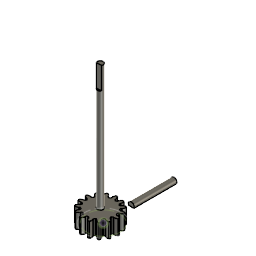
axle (Autodesk Fusion 360 design; units mm, degrees)
part number: 2026-05-16-01-15-47-219
Autodesk Fusion 360 part; units mm, degrees
note: some values were not read from the file. Chosen so that the rebuilt part matches the saved one: which bodies a step acts on; which pieces of a blend or face edit are solid. Set by a fixed rule: which sketch regions a step uses.
(part 1 of 4)
sketch "Sketch1" plane through (0, 0, 0) normal (0, 0, 1) x (1, 0, 0)
  circle A0 centre (0, 0) radius 12.5 construction
  dimension "d1" = 25
  constraint coincident A0.centre origin
  measures "d1" diameter of A0
sketch "Base Circle" plane through (0, 0, 0) normal (0, 0, 1) x (1, 0, 0)
  circle A0 centre (0, 0) radius 9.3279
  circle A1 centre (0, 0) radius 1.15
extrude "Extrude1" add sketch "Base Circle" along normal blind 10 makes body 1
sketch "Gear Tooth" plane through (0, 0, 0) normal (0, 0, 1) x (1, 0, 0)
  spline S0 degree 5 poles (10.2902, -1.2369) (10.2964, -1.2376) (10.3089, -1.2389) (10.3277, -1.2404) (10.3528, -1.2412) (10.3842, -1.2409) (10.4157, -1.2395) (10.4473, -1.2374) (10.4789, -1.2351) (10.5106, -1.2325) (10.5422, -1.2296) (10.5739, -1.2264) (10.6056, -1.2228) (10.6373, -1.2187) (10.6691, -1.2141) (10.7008, -1.209) (10.7326, -1.2035) (10.7644, -1.1976) (10.7962, -1.1915) (10.828, -1.1851) (10.8597, -1.1784) (10.8915, -1.1714) (10.9233, -1.1641) (10.9551, -1.1564) (10.9869, -1.1485) (11.0187, -1.1402) (11.0505, -1.1317) (11.0823, -1.1229) (11.114, -1.1138) (11.1458, -1.1044) (11.1776, -1.0948) (11.2093, -1.085) (11.241, -1.0748) (11.2727, -1.0645) (11.3045, -1.0538) (11.3361, -1.0429) (11.3678, -1.0318) (11.3995, -1.0204) (11.4311, -1.0087) (11.4627, -0.9969) (11.4943, -0.9847) (11.5259, -0.9724) (11.5575, -0.9598) (11.589, -0.947) (11.6206, -0.934) (11.6521, -0.9207) (11.6835, -0.9072) (11.715, -0.8935) (11.7464, -0.8796) (11.7778, -0.8654) (11.8091, -0.8511) (11.8405, -0.8365) (11.8718, -0.8217) (11.9031, -0.8067) (11.9343, -0.7914) (11.9655, -0.776) (11.9967, -0.7603) (12.0279, -0.7445) (12.059, -0.7284) (12.0901, -0.7122) (12.1211, -0.6957) (12.1521, -0.679) (12.1831, -0.6622) (12.214, -0.6451) (12.2449, -0.6278) (12.2758, -0.6103) (12.3066, -0.5927) (12.3374, -0.5748) (12.3682, -0.5567) (12.3988, -0.5385) (12.4295, -0.52) (12.454, -0.5051) (12.4723, -0.4939) (12.4846, -0.4863) (12.4907, -0.4825) knots 0 0 0 0 0 0 0.01428571 0.02857143 0.04285714 0.05714286 0.07142857 0.08571429 0.1 0.11428571 0.12857143 0.14285714 0.15714286 0.17142857 0.18571429 0.2 0.21428571 0.22857143 0.24285714 0.25714286 0.27142857 0.28571429 0.3 0.31428571 0.32857143 0.34285714 0.35714286 0.37142857 0.38571429 0.4 0.41428571 0.42857143 0.44285714 0.45714286 0.47142857 0.48571429 0.5 0.51428571 0.52857143 0.54285714 0.55714286 0.57142857 0.58571429 0.6 0.61428571 0.62857143 0.64285714 0.65714286 0.67142857 0.68571429 0.7 0.71428571 0.72857143 0.74285714 0.75714286 0.77142857 0.78571429 0.8 0.81428571 0.82857143 0.84285714 0.85714286 0.87142857 0.88571429 0.9 0.91428571 0.92857143 0.94285714 0.95714286 0.97142857 0.98571429 1 1 1 1 1 1
  spline S1 degree 5 poles (10.2902, 1.2369) (10.2964, 1.2376) (10.3089, 1.2389) (10.3277, 1.2404) (10.3528, 1.2412) (10.3842, 1.2409) (10.4157, 1.2395) (10.4473, 1.2374) (10.4789, 1.2351) (10.5106, 1.2325) (10.5422, 1.2296) (10.5739, 1.2264) (10.6056, 1.2228) (10.6373, 1.2187) (10.6691, 1.2141) (10.7008, 1.209) (10.7326, 1.2035) (10.7644, 1.1976) (10.7962, 1.1915) (10.828, 1.1851) (10.8597, 1.1784) (10.8915, 1.1714) (10.9233, 1.1641) (10.9551, 1.1564) (10.9869, 1.1485) (11.0187, 1.1402) (11.0505, 1.1317) (11.0823, 1.1229) (11.114, 1.1138) (11.1458, 1.1044) (11.1776, 1.0948) (11.2093, 1.085) (11.241, 1.0748) (11.2727, 1.0645) (11.3045, 1.0538) (11.3361, 1.0429) (11.3678, 1.0318) (11.3995, 1.0204) (11.4311, 1.0087) (11.4627, 0.9969) (11.4943, 0.9847) (11.5259, 0.9724) (11.5575, 0.9598) (11.589, 0.947) (11.6206, 0.934) (11.6521, 0.9207) (11.6835, 0.9072) (11.715, 0.8935) (11.7464, 0.8796) (11.7778, 0.8654) (11.8091, 0.8511) (11.8405, 0.8365) (11.8718, 0.8217) (11.9031, 0.8067) (11.9343, 0.7914) (11.9655, 0.776) (11.9967, 0.7603) (12.0279, 0.7445) (12.059, 0.7284) (12.0901, 0.7122) (12.1211, 0.6957) (12.1521, 0.679) (12.1831, 0.6622) (12.214, 0.6451) (12.2449, 0.6278) (12.2758, 0.6103) (12.3066, 0.5927) (12.3374, 0.5748) (12.3682, 0.5567) (12.3988, 0.5385) (12.4295, 0.52) (12.454, 0.5051) (12.4723, 0.4939) (12.4846, 0.4863) (12.4907, 0.4825) knots 0 0 0 0 0 0 0.01428571 0.02857143 0.04285714 0.05714286 0.07142857 0.08571429 0.1 0.11428571 0.12857143 0.14285714 0.15714286 0.17142857 0.18571429 0.2 0.21428571 0.22857143 0.24285714 0.25714286 0.27142857 0.28571429 0.3 0.31428571 0.32857143 0.34285714 0.35714286 0.37142857 0.38571429 0.4 0.41428571 0.42857143 0.44285714 0.45714286 0.47142857 0.48571429 0.5 0.51428571 0.52857143 0.54285714 0.55714286 0.57142857 0.58571429 0.6 0.61428571 0.62857143 0.64285714 0.65714286 0.67142857 0.68571429 0.7 0.71428571 0.72857143 0.74285714 0.75714286 0.77142857 0.78571429 0.8 0.81428571 0.82857143 0.84285714 0.85714286 0.87142857 0.88571429 0.9 0.91428571 0.92857143 0.94285714 0.95714286 0.97142857 0.98571429 1 1 1 1 1 1
  arc A0 (12.4907, -0.4825) -> (12.4907, 0.4825) centre (0, 0) ccw
  line L0 (9.2514, -1.112) -> (10.2902, -1.2369)
  line L1 (9.2514, 1.112) -> (10.2902, 1.2369)
  line L2 (9.2514, -1.112) -> (9.2514, 1.112)
  point P0 (10.4437, -1.2376)
  point P1 (10.599, -1.2235)
  point P2 (10.7553, -1.1992)
  point P3 (10.9123, -1.1666)
  point P4 (11.0699, -1.1263)
  point P5 (11.2278, -1.079)
  point P6 (11.3861, -1.0252)
  point P7 (11.5444, -0.965)
  point P8 (11.7028, -0.8988)
  point P9 (11.861, -0.8267)
  point P10 (12.019, -0.749)
  point P11 (12.1767, -0.6656)
  point P12 (12.334, -0.5768)
  point P13 (10.4437, 1.2376)
  point P14 (10.599, 1.2235)
  point P15 (10.7553, 1.1992)
  point P16 (10.9123, 1.1666)
  point P17 (11.0699, 1.1263)
  point P18 (11.2278, 1.079)
  point P19 (11.3861, 1.0252)
  point P20 (11.5444, 0.965)
  point P21 (11.7028, 0.8988)
  point P22 (11.861, 0.8267)
  point P23 (12.019, 0.749)
  point P24 (12.1767, 0.6656)
  point P25 (12.334, 0.5768)
extrude "Extrude2" add sketch "Gear Tooth" along normal blind 10 bodies 1
fillet "Fillet1" radius 0.8 2 edges at (9.2613, -1.1132, 5) (9.2613, 1.1132, 5) on bodies 1
pattern_circular "C-Pattern1" count 15 over 360 about axis through (0, 0, 0) along (0, 0, 1) of "Extrude2", "Fillet1"
sketch "Diametrial Pitch Circle" plane through (0, 0, 0) normal (0, 0, 1) x (1, 0, 0)
  circle A0 centre (0, 0) radius 11.0294 construction
sketch "Sketch5" plane through (0, 0, 0) normal (0, 0, 1) x (1, 0, 0)
  circle A0 centre (0, 0) radius 1.15
  dimension "d10" = 2.3
  constraint coincident A0.centre origin
  measures "d10" diameter of A0
extrude "Extrude3" add sketch "Sketch5" along normal blind 10 bodies 1
sketch "Sketch6" plane through (0, 0, 0) normal (0, 0, 1) x (1, 0, 0)
  circle A0 centre (0, 0) radius 2
  line L0 (1.7319, -1.0003) -> (-1.7676, -0.9358)
  dimension "d13" = 4
  dimension "d14" = 3.5
  constraint coincident A0.centre origin
  constraint coincident A0 L0.start
  constraint coincident A0 L0.end
  measures "d13" diameter of A0
  measures "d14" distance of L0.start L0.end
move_body "Move1" bodies 1 to x (1, 0, 0) y (0, 1, 0) z (0, 0, 1) at (0, 0, 80)
extrude "Extrude4" add sketch "Sketch6" along normal blind 80 bodies 1
extrude "Extrude5" cut sketch "Sketch6" along normal blind 15 contours A0 L0 picked at (-0.551, -1.0376) bodies 1
move_body "Move2" bodies 1 to x (1, 0, 0) y (0, -1, 0) z (0, 0, -1) at (0, 0.0546, 170)
extrude "Extrude6" add sketch "Sketch6" along normal blind 80 bodies 1
extrude "Extrude7" cut sketch "Sketch6" along normal blind 15 contours A0 L0 picked at (-0.551, -1.0376) bodies 1
move_body "Move3" bodies 1 to x (1, 0, 0) y (0, 0, 1) z (0, -1, 0) at (0, 0, 0)
move_body "Move4" bodies 1 to x (1, 0, 0) y (0, 1, 0) z (0, 0, 1) at (0, 85, 0)
move_body "Move5" bodies 1 to x (1, 0, 0) y (0, 1, 0) z (0, 0, 1) at (0, 0, 13)
sketch "Sketch7" plane through (0, 5, 0) normal (0, 1, 0) x (-1, 0, 0)
  circle A0 centre (0, 13) radius 2
  arc A1 (-9.1027, 15.0919) -> (-9.1444, 14.8959) centre (0, 13.0546) ccw
  arc A2 (-10.0241, 14.2595) -> (-9.1444, 14.8959) centre (-9.9287, 15.0538) ccw
  line L0 (-10.0241, 14.2595) -> (-10.2902, 14.2915)
  spline S0 degree 5 poles (-10.2902, 14.2915) (-10.2964, 14.2922) (-10.3089, 14.2935) (-10.3277, 14.295) (-10.3528, 14.2958) (-10.3842, 14.2955) (-10.4157, 14.2941) (-10.4473, 14.2921) (-10.4789, 14.2897) (-10.5106, 14.2871) (-10.5422, 14.2842) (-10.5739, 14.281) (-10.6056, 14.2774) (-10.6373, 14.2733) (-10.6691, 14.2687) (-10.7008, 14.2636) (-10.7326, 14.2581) (-10.7644, 14.2522) (-10.7962, 14.2461) (-10.828, 14.2397) (-10.8597, 14.233) (-10.8915, 14.226) (-10.9233, 14.2187) (-10.9551, 14.211) (-10.9869, 14.2031) (-11.0187, 14.1948) (-11.0505, 14.1863) (-11.0823, 14.1775) (-11.114, 14.1684) (-11.1458, 14.1591) (-11.1776, 14.1494) (-11.2093, 14.1396) (-11.241, 14.1295) (-11.2727, 14.1191) (-11.3045, 14.1084) (-11.3361, 14.0975) (-11.3678, 14.0864) (-11.3995, 14.075) (-11.4311, 14.0633) (-11.4627, 14.0515) (-11.4943, 14.0394) (-11.5259, 14.027) (-11.5575, 14.0144) (-11.589, 14.0016) (-11.6206, 13.9886) (-11.6521, 13.9753) (-11.6835, 13.9618) (-11.715, 13.9481) (-11.7464, 13.9342) (-11.7778, 13.92) (-11.8091, 13.9057) (-11.8405, 13.8911) (-11.8718, 13.8763) (-11.9031, 13.8613) (-11.9343, 13.846) (-11.9655, 13.8306) (-11.9967, 13.815) (-12.0279, 13.7991) (-12.059, 13.783) (-12.0901, 13.7668) (-12.1211, 13.7503) (-12.1521, 13.7336) (-12.1831, 13.7168) (-12.214, 13.6997) (-12.2449, 13.6824) (-12.2758, 13.6649) (-12.3066, 13.6473) (-12.3374, 13.6294) (-12.3682, 13.6113) (-12.3988, 13.5931) (-12.4295, 13.5746) (-12.454, 13.5597) (-12.4723, 13.5485) (-12.4846, 13.5409) (-12.4907, 13.5371) knots 0 0 0 0 0 0 0.01428571 0.02857143 0.04285714 0.05714286 0.07142857 0.08571429 0.1 0.11428571 0.12857143 0.14285714 0.15714286 0.17142857 0.18571429 0.2 0.21428571 0.22857143 0.24285714 0.25714286 0.27142857 0.28571429 0.3 0.31428571 0.32857143 0.34285714 0.35714286 0.37142857 0.38571429 0.4 0.41428571 0.42857143 0.44285714 0.45714286 0.47142857 0.48571429 0.5 0.51428571 0.52857143 0.54285714 0.55714286 0.57142857 0.58571429 0.6 0.61428571 0.62857143 0.64285714 0.65714286 0.67142857 0.68571429 0.7 0.71428571 0.72857143 0.74285714 0.75714286 0.77142857 0.78571429 0.8 0.81428571 0.82857143 0.84285714 0.85714286 0.87142857 0.88571429 0.9 0.91428571 0.92857143 0.94285714 0.95714286 0.97142857 0.98571429 1 1 1 1 1 1
  arc A3 (-12.4907, 13.5371) -> (-12.4907, 12.5721) centre (0, 13.0546) ccw
  spline S1 degree 5 poles (-12.4907, 12.5721) (-12.4846, 12.5683) (-12.4723, 12.5608) (-12.454, 12.5495) (-12.4295, 12.5346) (-12.3988, 12.5161) (-12.3682, 12.4979) (-12.3374, 12.4798) (-12.3066, 12.4619) (-12.2758, 12.4443) (-12.2449, 12.4268) (-12.214, 12.4095) (-12.1831, 12.3925) (-12.1521, 12.3756) (-12.1211, 12.3589) (-12.0901, 12.3424) (-12.059, 12.3262) (-12.0279, 12.3101) (-11.9967, 12.2943) (-11.9655, 12.2786) (-11.9343, 12.2632) (-11.9031, 12.2479) (-11.8718, 12.2329) (-11.8405, 12.2181) (-11.8091, 12.2035) (-11.7778, 12.1892) (-11.7464, 12.175) (-11.715, 12.1611) (-11.6835, 12.1474) (-11.6521, 12.1339) (-11.6206, 12.1206) (-11.589, 12.1076) (-11.5575, 12.0948) (-11.5259, 12.0822) (-11.4943, 12.0699) (-11.4627, 12.0578) (-11.4311, 12.0459) (-11.3995, 12.0342) (-11.3678, 12.0229) (-11.3361, 12.0117) (-11.3045, 12.0008) (-11.2727, 11.9902) (-11.241, 11.9798) (-11.2093, 11.9696) (-11.1776, 11.9598) (-11.1458, 11.9502) (-11.114, 11.9408) (-11.0823, 11.9317) (-11.0505, 11.9229) (-11.0187, 11.9144) (-10.9869, 11.9061) (-10.9551, 11.8982) (-10.9233, 11.8905) (-10.8915, 11.8832) (-10.8597, 11.8762) (-10.828, 11.8696) (-10.7962, 11.8631) (-10.7644, 11.857) (-10.7326, 11.8512) (-10.7008, 11.8457) (-10.6691, 11.8406) (-10.6373, 11.8359) (-10.6056, 11.8318) (-10.5739, 11.8282) (-10.5422, 11.825) (-10.5106, 11.8222) (-10.4789, 11.8195) (-10.4473, 11.8172) (-10.4157, 11.8151) (-10.3842, 11.8138) (-10.3528, 11.8134) (-10.3277, 11.8143) (-10.3089, 11.8157) (-10.2964, 11.817) (-10.2902, 11.8177) knots -1 -1 -1 -1 -1 -1 -0.98571429 -0.97142857 -0.95714286 -0.94285714 -0.92857143 -0.91428571 -0.9 -0.88571429 -0.87142857 -0.85714286 -0.84285714 -0.82857143 -0.81428571 -0.8 -0.78571429 -0.77142857 -0.75714286 -0.74285714 -0.72857143 -0.71428571 -0.7 -0.68571429 -0.67142857 -0.65714286 -0.64285714 -0.62857143 -0.61428571 -0.6 -0.58571429 -0.57142857 -0.55714286 -0.54285714 -0.52857143 -0.51428571 -0.5 -0.48571429 -0.47142857 -0.45714286 -0.44285714 -0.42857143 -0.41428571 -0.4 -0.38571429 -0.37142857 -0.35714286 -0.34285714 -0.32857143 -0.31428571 -0.3 -0.28571429 -0.27142857 -0.25714286 -0.24285714 -0.22857143 -0.21428571 -0.2 -0.18571429 -0.17142857 -0.15714286 -0.14285714 -0.12857143 -0.11428571 -0.1 -0.08571429 -0.07142857 -0.05714286 -0.04285714 -0.02857143 -0.01428571 0 0 0 0 0 0
  line L1 (-10.2902, 11.8177) -> (-10.0241, 11.8497)
  arc A4 (-9.1444, 11.2134) -> (-10.0241, 11.8497) centre (-9.9287, 11.0554) ccw
  arc A5 (-9.1444, 11.2134) -> (-9.1027, 11.0173) centre (0, 13.0546) ccw
  arc A6 (-9.6476, 10.0781) -> (-9.1027, 11.0173) centre (-9.8834, 10.8426) ccw
  line L2 (-9.6476, 10.0781) -> (-9.9036, 9.9991)
  spline S2 degree 5 poles (-9.9036, 9.9991) (-9.9096, 9.9973) (-9.9216, 9.9934) (-9.9393, 9.9871) (-9.9626, 9.9777) (-9.9912, 9.9645) (-10.0194, 9.9505) (-10.0474, 9.9358) (-10.0753, 9.9207) (-10.1032, 9.9055) (-10.1309, 9.89) (-10.1586, 9.8742) (-10.1861, 9.858) (-10.2134, 9.8413) (-10.2405, 9.8242) (-10.2674, 9.8066) (-10.2942, 9.7887) (-10.3209, 9.7704) (-10.3474, 9.7519) (-10.3738, 9.7331) (-10.4002, 9.714) (-10.4264, 9.6947) (-10.4524, 9.6751) (-10.4784, 9.6552) (-10.5042, 9.635) (-10.5299, 9.6146) (-10.5554, 9.5938) (-10.5809, 9.5728) (-10.6062, 9.5516) (-10.6314, 9.5302) (-10.6565, 9.5085) (-10.6815, 9.4865) (-10.7064, 9.4644) (-10.7311, 9.442) (-10.7558, 9.4194) (-10.7803, 9.3965) (-10.8047, 9.3735) (-10.829, 9.3502) (-10.8531, 9.3267) (-10.8772, 9.303) (-10.9011, 9.279) (-10.925, 9.2549) (-10.9487, 9.2306) (-10.9723, 9.2061) (-10.9958, 9.1813) (-11.0192, 9.1564) (-11.0424, 9.1313) (-11.0656, 9.106) (-11.0886, 9.0805) (-11.1115, 9.0548) (-11.1344, 9.0289) (-11.157, 9.0028) (-11.1796, 8.9766) (-11.2021, 8.9501) (-11.2244, 8.9235) (-11.2467, 8.8967) (-11.2688, 8.8697) (-11.2908, 8.8426) (-11.3127, 8.8152) (-11.3345, 8.7877) (-11.3562, 8.7601) (-11.3777, 8.7322) (-11.3991, 8.7042) (-11.4205, 8.676) (-11.4417, 8.6477) (-11.4628, 8.6192) (-11.4837, 8.5905) (-11.5046, 8.5616) (-11.5253, 8.5326) (-11.5459, 8.5035) (-11.5664, 8.4742) (-11.5827, 8.4506) (-11.5949, 8.4328) (-11.603, 8.4209) (-11.6071, 8.415) knots 0 0 0 0 0 0 0.01428571 0.02857143 0.04285714 0.05714286 0.07142857 0.08571429 0.1 0.11428571 0.12857143 0.14285714 0.15714286 0.17142857 0.18571429 0.2 0.21428571 0.22857143 0.24285714 0.25714286 0.27142857 0.28571429 0.3 0.31428571 0.32857143 0.34285714 0.35714286 0.37142857 0.38571429 0.4 0.41428571 0.42857143 0.44285714 0.45714286 0.47142857 0.48571429 0.5 0.51428571 0.52857143 0.54285714 0.55714286 0.57142857 0.58571429 0.6 0.61428571 0.62857143 0.64285714 0.65714286 0.67142857 0.68571429 0.7 0.71428571 0.72857143 0.74285714 0.75714286 0.77142857 0.78571429 0.8 0.81428571 0.82857143 0.84285714 0.85714286 0.87142857 0.88571429 0.9 0.91428571 0.92857143 0.94285714 0.95714286 0.97142857 0.98571429 1 1 1 1 1 1
  arc A7 (-11.6071, 8.415) -> (-11.2145, 7.5334) centre (0, 13.0546) ccw
  spline S3 degree 5 poles (-11.2145, 7.5334) (-11.2074, 7.5324) (-11.1932, 7.5305) (-11.1718, 7.5277) (-11.1434, 7.524) (-11.1079, 7.5196) (-11.0724, 7.5154) (-11.037, 7.5114) (-11.0016, 7.5076) (-10.9663, 7.504) (-10.931, 7.5006) (-10.8957, 7.4974) (-10.8605, 7.4944) (-10.8253, 7.4916) (-10.7902, 7.489) (-10.7552, 7.4865) (-10.7202, 7.4843) (-10.6852, 7.4823) (-10.6503, 7.4805) (-10.6154, 7.4789) (-10.5806, 7.4775) (-10.5459, 7.4763) (-10.5112, 7.4753) (-10.4766, 7.4745) (-10.442, 7.4739) (-10.4075, 7.4735) (-10.3731, 7.4734) (-10.3387, 7.4734) (-10.3044, 7.4737) (-10.2702, 7.4742) (-10.236, 7.4749) (-10.2019, 7.4758) (-10.1679, 7.4769) (-10.134, 7.4783) (-10.1001, 7.4798) (-10.0663, 7.4816) (-10.0326, 7.4836) (-9.9989, 7.4859) (-9.9654, 7.4883) (-9.9319, 7.491) (-9.8985, 7.494) (-9.8652, 7.4971) (-9.832, 7.5006) (-9.7989, 7.5042) (-9.7659, 7.5081) (-9.733, 7.5122) (-9.7002, 7.5166) (-9.6674, 7.5212) (-9.6348, 7.5261) (-9.6023, 7.5312) (-9.5699, 7.5366) (-9.5376, 7.5423) (-9.5055, 7.5483) (-9.4735, 7.5545) (-9.4416, 7.5611) (-9.4098, 7.5679) (-9.3782, 7.5749) (-9.3466, 7.5823) (-9.3152, 7.5899) (-9.284, 7.5977) (-9.2529, 7.606) (-9.222, 7.6147) (-9.1914, 7.6238) (-9.1609, 7.6334) (-9.1307, 7.6434) (-9.1006, 7.6537) (-9.0706, 7.6642) (-9.0408, 7.6748) (-9.0111, 7.6858) (-8.9818, 7.6974) (-8.9529, 7.7099) (-8.9303, 7.7208) (-8.9137, 7.7298) (-8.9029, 7.7361) (-8.8975, 7.7393) knots -1 -1 -1 -1 -1 -1 -0.98571429 -0.97142857 -0.95714286 -0.94285714 -0.92857143 -0.91428571 -0.9 -0.88571429 -0.87142857 -0.85714286 -0.84285714 -0.82857143 -0.81428571 -0.8 -0.78571429 -0.77142857 -0.75714286 -0.74285714 -0.72857143 -0.71428571 -0.7 -0.68571429 -0.67142857 -0.65714286 -0.64285714 -0.62857143 -0.61428571 -0.6 -0.58571429 -0.57142857 -0.55714286 -0.54285714 -0.52857143 -0.51428571 -0.5 -0.48571429 -0.47142857 -0.45714286 -0.44285714 -0.42857143 -0.41428571 -0.4 -0.38571429 -0.37142857 -0.35714286 -0.34285714 -0.32857143 -0.31428571 -0.3 -0.28571429 -0.27142857 -0.25714286 -0.24285714 -0.22857143 -0.21428571 -0.2 -0.18571429 -0.17142857 -0.15714286 -0.14285714 -0.12857143 -0.11428571 -0.1 -0.08571429 -0.07142857 -0.05714286 -0.04285714 -0.02857143 -0.01428571 0 0 0 0 0 0
  line L3 (-8.8975, 7.7393) -> (-8.6674, 7.8767)
  arc A8 (-7.6049, 7.6532) -> (-8.6674, 7.8767) centre (-8.2572, 7.1899) ccw
  arc A9 (-7.6049, 7.6532) -> (-7.4871, 7.491) centre (0, 13.0546) ccw
  arc A10 (-7.6029, 6.4114) -> (-7.4871, 7.491) centre (-8.1292, 7.0139) ccw
  line L4 (-7.6029, 6.4114) -> (-7.8046, 6.2351)
  spline S4 degree 5 poles (-7.8046, 6.2351) (-7.8094, 6.231) (-7.8187, 6.2226) (-7.8323, 6.2096) (-7.8498, 6.1915) (-7.8705, 6.1679) (-7.8906, 6.1436) (-7.9102, 6.1187) (-7.9296, 6.0937) (-7.9488, 6.0684) (-7.9679, 6.043) (-7.9867, 6.0173) (-8.0053, 5.9913) (-8.0234, 5.965) (-8.0412, 5.9383) (-8.0587, 5.9113) (-8.0759, 5.884) (-8.0928, 5.8565) (-8.1095, 5.8287) (-8.126, 5.8008) (-8.1423, 5.7727) (-8.1584, 5.7444) (-8.1742, 5.7159) (-8.1898, 5.6872) (-8.2052, 5.6582) (-8.2203, 5.6291) (-8.2352, 5.5997) (-8.2499, 5.5702) (-8.2645, 5.5405) (-8.2788, 5.5107) (-8.2929, 5.4807) (-8.3068, 5.4505) (-8.3205, 5.4201) (-8.334, 5.3896) (-8.3473, 5.3589) (-8.3604, 5.3281) (-8.3733, 5.2971) (-8.386, 5.2659) (-8.3985, 5.2346) (-8.4109, 5.2032) (-8.423, 5.1716) (-8.435, 5.1398) (-8.4468, 5.108) (-8.4584, 5.076) (-8.4698, 5.0438) (-8.481, 5.0115) (-8.492, 4.9791) (-8.5029, 4.9466) (-8.5135, 4.9139) (-8.524, 4.8811) (-8.5343, 4.8482) (-8.5445, 4.8151) (-8.5544, 4.782) (-8.5642, 4.7487) (-8.5738, 4.7153) (-8.5832, 4.6817) (-8.5924, 4.6481) (-8.6015, 4.6143) (-8.6104, 4.5805) (-8.6191, 4.5465) (-8.6276, 4.5124) (-8.636, 4.4782) (-8.6442, 4.4439) (-8.6522, 4.4094) (-8.66, 4.3749) (-8.6677, 4.3403) (-8.6752, 4.3056) (-8.6825, 4.2707) (-8.6896, 4.2358) (-8.6966, 4.2008) (-8.7034, 4.1657) (-8.7087, 4.1375) (-8.7126, 4.1163) (-8.7152, 4.1022) (-8.7165, 4.0951) knots 0 0 0 0 0 0 0.01428571 0.02857143 0.04285714 0.05714286 0.07142857 0.08571429 0.1 0.11428571 0.12857143 0.14285714 0.15714286 0.17142857 0.18571429 0.2 0.21428571 0.22857143 0.24285714 0.25714286 0.27142857 0.28571429 0.3 0.31428571 0.32857143 0.34285714 0.35714286 0.37142857 0.38571429 0.4 0.41428571 0.42857143 0.44285714 0.45714286 0.47142857 0.48571429 0.5 0.51428571 0.52857143 0.54285714 0.55714286 0.57142857 0.58571429 0.6 0.61428571 0.62857143 0.64285714 0.65714286 0.67142857 0.68571429 0.7 0.71428571 0.72857143 0.74285714 0.75714286 0.77142857 0.78571429 0.8 0.81428571 0.82857143 0.84285714 0.85714286 0.87142857 0.88571429 0.9 0.91428571 0.92857143 0.94285714 0.95714286 0.97142857 0.98571429 1 1 1 1 1 1
  arc A11 (-8.7165, 4.0951) -> (-7.9993, 3.4494) centre (0, 13.0546) ccw
  spline S5 degree 5 poles (-7.9993, 3.4494) (-7.9924, 3.4514) (-7.9786, 3.4554) (-7.958, 3.4615) (-7.9305, 3.4697) (-7.8963, 3.4802) (-7.8622, 3.4908) (-7.8282, 3.5015) (-7.7943, 3.5124) (-7.7606, 3.5235) (-7.7269, 3.5348) (-7.6934, 3.5462) (-7.66, 3.5577) (-7.6267, 3.5695) (-7.5936, 3.5813) (-7.5606, 3.5934) (-7.5277, 3.6056) (-7.495, 3.618) (-7.4623, 3.6305) (-7.4298, 3.6432) (-7.3975, 3.6561) (-7.3652, 3.6691) (-7.3332, 3.6823) (-7.3012, 3.6957) (-7.2694, 3.7092) (-7.2377, 3.7229) (-7.2062, 3.7368) (-7.1748, 3.7508) (-7.1436, 3.765) (-7.1125, 3.7794) (-7.0816, 3.7939) (-7.0508, 3.8086) (-7.0202, 3.8235) (-6.9897, 3.8385) (-6.9594, 3.8537) (-6.9293, 3.8691) (-6.8993, 3.8847) (-6.8695, 3.9004) (-6.8398, 3.9163) (-6.8103, 3.9324) (-6.781, 3.9486) (-6.7519, 3.9651) (-6.723, 3.9817) (-6.6942, 3.9985) (-6.6656, 4.0155) (-6.6372, 4.0326) (-6.609, 4.05) (-6.581, 4.0675) (-6.5532, 4.0852) (-6.5256, 4.1031) (-6.4982, 4.1212) (-6.471, 4.1396) (-6.4441, 4.1581) (-6.4174, 4.1768) (-6.3909, 4.1958) (-6.3646, 4.2149) (-6.3386, 4.2342) (-6.3128, 4.2538) (-6.2872, 4.2735) (-6.2618, 4.2934) (-6.2368, 4.3136) (-6.2121, 4.3341) (-6.1878, 4.3549) (-6.1639, 4.376) (-6.1404, 4.3974) (-6.1171, 4.4191) (-6.0939, 4.4408) (-6.071, 4.4627) (-6.0484, 4.4848) (-6.0263, 4.5073) (-6.005, 4.5305) (-5.9888, 4.5497) (-5.9773, 4.5646) (-5.9699, 4.5747) (-5.9663, 4.5799) knots -1 -1 -1 -1 -1 -1 -0.98571429 -0.97142857 -0.95714286 -0.94285714 -0.92857143 -0.91428571 -0.9 -0.88571429 -0.87142857 -0.85714286 -0.84285714 -0.82857143 -0.81428571 -0.8 -0.78571429 -0.77142857 -0.75714286 -0.74285714 -0.72857143 -0.71428571 -0.7 -0.68571429 -0.67142857 -0.65714286 -0.64285714 -0.62857143 -0.61428571 -0.6 -0.58571429 -0.57142857 -0.55714286 -0.54285714 -0.52857143 -0.51428571 -0.5 -0.48571429 -0.47142857 -0.45714286 -0.44285714 -0.42857143 -0.41428571 -0.4 -0.38571429 -0.37142857 -0.35714286 -0.34285714 -0.32857143 -0.31428571 -0.3 -0.28571429 -0.27142857 -0.25714286 -0.24285714 -0.22857143 -0.21428571 -0.2 -0.18571429 -0.17142857 -0.15714286 -0.14285714 -0.12857143 -0.11428571 -0.1 -0.08571429 -0.07142857 -0.05714286 -0.04285714 -0.02857143 -0.01428571 0 0 0 0 0 0
  line L5 (-5.9663, 4.5799) -> (-5.8121, 4.799)
  arc A12 (-4.7505, 5.0269) -> (-5.8121, 4.799) centre (-5.1579, 4.3385) ccw
  arc A13 (-4.7505, 5.0269) -> (-4.5769, 4.9267) centre (0, 13.0546) ccw
  arc A14 (-4.2435, 3.8934) -> (-4.5769, 4.9267) centre (-4.9694, 4.2297) ccw
  line L6 (-4.2435, 3.8934) -> (-4.3562, 3.6503)
  spline S6 degree 5 poles (-4.3562, 3.6503) (-4.3588, 3.6446) (-4.3639, 3.6331) (-4.3711, 3.6157) (-4.3796, 3.5921) (-4.389, 3.5621) (-4.3974, 3.5317) (-4.4053, 3.501) (-4.4128, 3.4702) (-4.4201, 3.4393) (-4.4271, 3.4083) (-4.4339, 3.3772) (-4.4403, 3.3459) (-4.4461, 3.3145) (-4.4516, 3.2829) (-4.4565, 3.2511) (-4.4611, 3.2192) (-4.4654, 3.1872) (-4.4694, 3.155) (-4.4731, 3.1228) (-4.4765, 3.0905) (-4.4797, 3.0581) (-4.4826, 3.0256) (-4.4852, 2.993) (-4.4874, 2.9603) (-4.4894, 2.9276) (-4.4911, 2.8947) (-4.4925, 2.8617) (-4.4937, 2.8287) (-4.4946, 2.7956) (-4.4953, 2.7624) (-4.4957, 2.7292) (-4.4959, 2.6959) (-4.4958, 2.6625) (-4.4955, 2.6291) (-4.4949, 2.5956) (-4.4941, 2.562) (-4.4931, 2.5284) (-4.4918, 2.4947) (-4.4903, 2.4609) (-4.4885, 2.4271) (-4.4865, 2.3933) (-4.4843, 2.3594) (-4.4819, 2.3254) (-4.4792, 2.2914) (-4.4763, 2.2574) (-4.4732, 2.2233) (-4.4699, 2.1891) (-4.4664, 2.1549) (-4.4626, 2.1207) (-4.4586, 2.0864) (-4.4544, 2.0521) (-4.45, 2.0178) (-4.4454, 1.9834) (-4.4406, 1.949) (-4.4356, 1.9145) (-4.4303, 1.88) (-4.4249, 1.8455) (-4.4192, 1.8109) (-4.4133, 1.7763) (-4.4073, 1.7417) (-4.401, 1.7071) (-4.3945, 1.6724) (-4.3879, 1.6377) (-4.381, 1.603) (-4.3739, 1.5682) (-4.3666, 1.5335) (-4.3591, 1.4987) (-4.3515, 1.4638) (-4.3436, 1.429) (-4.3355, 1.3941) (-4.3289, 1.3662) (-4.3239, 1.3453) (-4.3205, 1.3314) (-4.3187, 1.3244) knots 0 0 0 0 0 0 0.01428571 0.02857143 0.04285714 0.05714286 0.07142857 0.08571429 0.1 0.11428571 0.12857143 0.14285714 0.15714286 0.17142857 0.18571429 0.2 0.21428571 0.22857143 0.24285714 0.25714286 0.27142857 0.28571429 0.3 0.31428571 0.32857143 0.34285714 0.35714286 0.37142857 0.38571429 0.4 0.41428571 0.42857143 0.44285714 0.45714286 0.47142857 0.48571429 0.5 0.51428571 0.52857143 0.54285714 0.55714286 0.57142857 0.58571429 0.6 0.61428571 0.62857143 0.64285714 0.65714286 0.67142857 0.68571429 0.7 0.71428571 0.72857143 0.74285714 0.75714286 0.77142857 0.78571429 0.8 0.81428571 0.82857143 0.84285714 0.85714286 0.87142857 0.88571429 0.9 0.91428571 0.92857143 0.94285714 0.95714286 0.97142857 0.98571429 1 1 1 1 1 1
  arc A15 (-4.3187, 1.3244) -> (-3.4009, 1.0262) centre (0, 13.0546) ccw
  spline S7 degree 5 poles (-3.4009, 1.0262) (-3.3954, 1.0308) (-3.3845, 1.0401) (-3.3681, 1.0541) (-3.3463, 1.0727) (-3.3193, 1.0962) (-3.2925, 1.1198) (-3.2658, 1.1434) (-3.2393, 1.1672) (-3.213, 1.191) (-3.1868, 1.215) (-3.1608, 1.239) (-3.135, 1.2632) (-3.1094, 1.2874) (-3.084, 1.3118) (-3.0587, 1.3362) (-3.0337, 1.3607) (-3.0088, 1.3854) (-2.9841, 1.4101) (-2.9595, 1.4349) (-2.9352, 1.4598) (-2.9111, 1.4848) (-2.8871, 1.5099) (-2.8634, 1.5352) (-2.8398, 1.5604) (-2.8165, 1.5858) (-2.7933, 1.6113) (-2.7703, 1.6369) (-2.7476, 1.6626) (-2.725, 1.6883) (-2.7027, 1.7142) (-2.6805, 1.7401) (-2.6586, 1.7662) (-2.6369, 1.7923) (-2.6154, 1.8185) (-2.5941, 1.8448) (-2.5731, 1.8713) (-2.5522, 1.8977) (-2.5316, 1.9243) (-2.5112, 1.951) (-2.491, 1.9778) (-2.4711, 2.0047) (-2.4514, 2.0316) (-2.432, 2.0587) (-2.4128, 2.0858) (-2.3939, 2.113) (-2.3751, 2.1403) (-2.3567, 2.1678) (-2.3385, 2.1953) (-2.3205, 2.2228) (-2.3029, 2.2505) (-2.2855, 2.2783) (-2.2684, 2.3062) (-2.2516, 2.3342) (-2.2352, 2.3622) (-2.219, 2.3904) (-2.203, 2.4187) (-2.1874, 2.447) (-2.172, 2.4754) (-2.157, 2.5039) (-2.1423, 2.5326) (-2.1281, 2.5613) (-2.1144, 2.5902) (-2.1011, 2.6192) (-2.0883, 2.6484) (-2.0758, 2.6776) (-2.0636, 2.7069) (-2.0515, 2.7362) (-2.0398, 2.7656) (-2.0288, 2.7952) (-2.0187, 2.825) (-2.0118, 2.8491) (-2.0073, 2.8674) (-2.0047, 2.8797) (-2.0035, 2.8858) knots -1 -1 -1 -1 -1 -1 -0.98571429 -0.97142857 -0.95714286 -0.94285714 -0.92857143 -0.91428571 -0.9 -0.88571429 -0.87142857 -0.85714286 -0.84285714 -0.82857143 -0.81428571 -0.8 -0.78571429 -0.77142857 -0.75714286 -0.74285714 -0.72857143 -0.71428571 -0.7 -0.68571429 -0.67142857 -0.65714286 -0.64285714 -0.62857143 -0.61428571 -0.6 -0.58571429 -0.57142857 -0.55714286 -0.54285714 -0.52857143 -0.51428571 -0.5 -0.48571429 -0.47142857 -0.45714286 -0.44285714 -0.42857143 -0.41428571 -0.4 -0.38571429 -0.37142857 -0.35714286 -0.34285714 -0.32857143 -0.31428571 -0.3 -0.28571429 -0.27142857 -0.25714286 -0.24285714 -0.22857143 -0.21428571 -0.2 -0.18571429 -0.17142857 -0.15714286 -0.14285714 -0.12857143 -0.11428571 -0.1 -0.08571429 -0.07142857 -0.05714286 -0.04285714 -0.02857143 -0.01428571 0 0 0 0 0 0
  line L7 (-2.0035, 2.8858) -> (-1.9517, 3.1488)
  arc A16 (-1.0746, 3.7888) -> (-1.9517, 3.1488) centre (-1.1668, 2.9941) ccw
  arc A17 (-1.0746, 3.7888) -> (-0.8753, 3.7678) centre (0, 13.0546) ccw
  arc A18 (-0.1505, 2.9594) -> (-0.8753, 3.7678) centre (-0.9504, 2.9714) ccw
  line L8 (-0.1505, 2.9594) -> (-0.1545, 2.6915)
  spline S8 degree 5 poles (-0.1545, 2.6915) (-0.1546, 2.6852) (-0.1546, 2.6727) (-0.154, 2.6538) (-0.1523, 2.6288) (-0.1486, 2.5976) (-0.1439, 2.5664) (-0.1386, 2.5352) (-0.133, 2.504) (-0.127, 2.4728) (-0.1209, 2.4416) (-0.1144, 2.4104) (-0.1075, 2.3793) (-0.1001, 2.3482) (-0.0922, 2.3171) (-0.0838, 2.286) (-0.075, 2.255) (-0.0659, 2.224) (-0.0564, 2.193) (-0.0467, 2.1621) (-0.0368, 2.1312) (-0.0265, 2.1003) (-0.0159, 2.0694) (-0.005, 2.0386) (0.0062, 2.0078) (0.0178, 1.9771) (0.0296, 1.9464) (0.0417, 1.9157) (0.054, 1.885) (0.0667, 1.8544) (0.0795, 1.8238) (0.0927, 1.7933) (0.1061, 1.7628) (0.1197, 1.7323) (0.1336, 1.7019) (0.1478, 1.6716) (0.1622, 1.6412) (0.1768, 1.6109) (0.1917, 1.5807) (0.2068, 1.5505) (0.2221, 1.5203) (0.2377, 1.4902) (0.2535, 1.4601) (0.2695, 1.4301) (0.2858, 1.4001) (0.3023, 1.3701) (0.319, 1.3403) (0.3359, 1.3104) (0.3531, 1.2806) (0.3704, 1.2509) (0.388, 1.2212) (0.4058, 1.1916) (0.4238, 1.162) (0.442, 1.1324) (0.4604, 1.1029) (0.479, 1.0735) (0.4978, 1.0441) (0.5168, 1.0148) (0.5361, 0.9855) (0.5555, 0.9563) (0.5751, 0.9272) (0.5949, 0.8981) (0.615, 0.869) (0.6352, 0.84) (0.6556, 0.8111) (0.6762, 0.7823) (0.697, 0.7534) (0.718, 0.7247) (0.7391, 0.696) (0.7605, 0.6674) (0.782, 0.6388) (0.7994, 0.616) (0.8126, 0.599) (0.8214, 0.5876) (0.8258, 0.5819) knots 0 0 0 0 0 0 0.01428571 0.02857143 0.04285714 0.05714286 0.07142857 0.08571429 0.1 0.11428571 0.12857143 0.14285714 0.15714286 0.17142857 0.18571429 0.2 0.21428571 0.22857143 0.24285714 0.25714286 0.27142857 0.28571429 0.3 0.31428571 0.32857143 0.34285714 0.35714286 0.37142857 0.38571429 0.4 0.41428571 0.42857143 0.44285714 0.45714286 0.47142857 0.48571429 0.5 0.51428571 0.52857143 0.54285714 0.55714286 0.57142857 0.58571429 0.6 0.61428571 0.62857143 0.64285714 0.65714286 0.67142857 0.68571429 0.7 0.71428571 0.72857143 0.74285714 0.75714286 0.77142857 0.78571429 0.8 0.81428571 0.82857143 0.84285714 0.85714286 0.87142857 0.88571429 0.9 0.91428571 0.92857143 0.94285714 0.95714286 0.97142857 0.98571429 1 1 1 1 1 1
  arc A19 (0.8258, 0.5819) -> (1.7855, 0.6828) centre (0, 13.0546) ccw
  spline S9 degree 5 poles (1.7855, 0.6828) (1.7886, 0.6893) (1.7949, 0.7022) (1.8042, 0.7216) (1.8164, 0.7476) (1.8316, 0.78) (1.8465, 0.8124) (1.8613, 0.8449) (1.8758, 0.8773) (1.8902, 0.9098) (1.9043, 0.9424) (1.9183, 0.9749) (1.932, 1.0075) (1.9455, 1.04) (1.9589, 1.0726) (1.972, 1.1052) (1.985, 1.1378) (1.9977, 1.1704) (2.0102, 1.2031) (2.0225, 1.2357) (2.0346, 1.2684) (2.0465, 1.3011) (2.0581, 1.3337) (2.0696, 1.3664) (2.0808, 1.3991) (2.0918, 1.4318) (2.1026, 1.4645) (2.1132, 1.4972) (2.1235, 1.5299) (2.1336, 1.5626) (2.1435, 1.5953) (2.1532, 1.628) (2.1627, 1.6608) (2.1719, 1.6935) (2.1808, 1.7262) (2.1896, 1.7589) (2.1981, 1.7915) (2.2063, 1.8242) (2.2144, 1.8569) (2.2221, 1.8896) (2.2297, 1.9222) (2.2369, 1.9549) (2.244, 1.9875) (2.2507, 2.0201) (2.2572, 2.0527) (2.2634, 2.0853) (2.2694, 2.1179) (2.2751, 2.1504) (2.2806, 2.1829) (2.2858, 2.2155) (2.2906, 2.2479) (2.2952, 2.2804) (2.2995, 2.3128) (2.3034, 2.3452) (2.3071, 2.3775) (2.3104, 2.4098) (2.3135, 2.4421) (2.3162, 2.4744) (2.3187, 2.5066) (2.3209, 2.5388) (2.3226, 2.5709) (2.3239, 2.6029) (2.3247, 2.6349) (2.325, 2.6668) (2.3248, 2.6987) (2.3244, 2.7304) (2.3236, 2.7622) (2.3227, 2.7939) (2.3214, 2.8255) (2.3195, 2.857) (2.3166, 2.8883) (2.3131, 2.9132) (2.3097, 2.9317) (2.3071, 2.944) (2.3057, 2.9501) knots -1 -1 -1 -1 -1 -1 -0.98571429 -0.97142857 -0.95714286 -0.94285714 -0.92857143 -0.91428571 -0.9 -0.88571429 -0.87142857 -0.85714286 -0.84285714 -0.82857143 -0.81428571 -0.8 -0.78571429 -0.77142857 -0.75714286 -0.74285714 -0.72857143 -0.71428571 -0.7 -0.68571429 -0.67142857 -0.65714286 -0.64285714 -0.62857143 -0.61428571 -0.6 -0.58571429 -0.57142857 -0.55714286 -0.54285714 -0.52857143 -0.51428571 -0.5 -0.48571429 -0.47142857 -0.45714286 -0.44285714 -0.42857143 -0.41428571 -0.4 -0.38571429 -0.37142857 -0.35714286 -0.34285714 -0.32857143 -0.31428571 -0.3 -0.28571429 -0.27142857 -0.25714286 -0.24285714 -0.22857143 -0.21428571 -0.2 -0.18571429 -0.17142857 -0.15714286 -0.14285714 -0.12857143 -0.11428571 -0.1 -0.08571429 -0.07142857 -0.05714286 -0.04285714 -0.02857143 -0.01428571 0 0 0 0 0 0
  line L9 (2.3057, 2.9501) -> (2.2461, 3.2113)
  arc A20 (2.787, 4.1528) -> (2.2461, 3.2113) centre (3.026, 3.3893) ccw
  arc A21 (2.787, 4.1528) -> (2.9776, 4.2147) centre (0, 13.0546) ccw
  arc A22 (3.9686, 3.771) -> (2.9776, 4.2147) centre (3.233, 3.4565) ccw
  line L10 (3.9686, 3.771) -> (4.0739, 3.5246)
  spline S10 degree 5 poles (4.0739, 3.5246) (4.0764, 3.5188) (4.0815, 3.5074) (4.0897, 3.4904) (4.1015, 3.4682) (4.1175, 3.4412) (4.1345, 3.4146) (4.152, 3.3882) (4.1699, 3.3621) (4.188, 3.336) (4.2063, 3.31) (4.2249, 3.2841) (4.2438, 3.2585) (4.2633, 3.2331) (4.2831, 3.2079) (4.3034, 3.1829) (4.3241, 3.1582) (4.345, 3.1336) (4.3662, 3.1091) (4.3877, 3.0848) (4.4094, 3.0606) (4.4313, 3.0366) (4.4536, 3.0127) (4.4761, 2.989) (4.4988, 2.9654) (4.5219, 2.942) (4.5452, 2.9188) (4.5687, 2.8956) (4.5924, 2.8727) (4.6164, 2.8498) (4.6406, 2.8271) (4.665, 2.8046) (4.6897, 2.7822) (4.7145, 2.7599) (4.7396, 2.7378) (4.7649, 2.7158) (4.7904, 2.6939) (4.8161, 2.6722) (4.842, 2.6506) (4.8681, 2.6292) (4.8944, 2.6078) (4.9208, 2.5867) (4.9475, 2.5656) (4.9744, 2.5447) (5.0014, 2.5239) (5.0287, 2.5033) (5.0561, 2.4828) (5.0837, 2.4624) (5.1115, 2.4421) (5.1394, 2.422) (5.1675, 2.4021) (5.1958, 2.3822) (5.2243, 2.3625) (5.2529, 2.3429) (5.2818, 2.3235) (5.3107, 2.3042) (5.3399, 2.285) (5.3692, 2.2659) (5.3987, 2.247) (5.4283, 2.2282) (5.4581, 2.2096) (5.488, 2.191) (5.5181, 2.1727) (5.5484, 2.1544) (5.5788, 2.1363) (5.6093, 2.1183) (5.6401, 2.1004) (5.6709, 2.0827) (5.7019, 2.0651) (5.7331, 2.0476) (5.7644, 2.0303) (5.7895, 2.0166) (5.8085, 2.0063) (5.8211, 1.9995) (5.8275, 1.9961) knots 0 0 0 0 0 0 0.01428571 0.02857143 0.04285714 0.05714286 0.07142857 0.08571429 0.1 0.11428571 0.12857143 0.14285714 0.15714286 0.17142857 0.18571429 0.2 0.21428571 0.22857143 0.24285714 0.25714286 0.27142857 0.28571429 0.3 0.31428571 0.32857143 0.34285714 0.35714286 0.37142857 0.38571429 0.4 0.41428571 0.42857143 0.44285714 0.45714286 0.47142857 0.48571429 0.5 0.51428571 0.52857143 0.54285714 0.55714286 0.57142857 0.58571429 0.6 0.61428571 0.62857143 0.64285714 0.65714286 0.67142857 0.68571429 0.7 0.71428571 0.72857143 0.74285714 0.75714286 0.77142857 0.78571429 0.8 0.81428571 0.82857143 0.84285714 0.85714286 0.87142857 0.88571429 0.9 0.91428571 0.92857143 0.94285714 0.95714286 0.97142857 0.98571429 1 1 1 1 1 1
  arc A23 (5.8275, 1.9961) -> (6.6632, 2.4786) centre (0, 13.0546) ccw
  spline S11 degree 5 poles (6.6632, 2.4786) (6.6634, 2.4858) (6.6639, 2.5002) (6.6645, 2.5217) (6.6651, 2.5504) (6.6658, 2.5861) (6.6662, 2.6218) (6.6665, 2.6575) (6.6666, 2.6931) (6.6665, 2.7286) (6.6662, 2.7641) (6.6657, 2.7995) (6.665, 2.8348) (6.6641, 2.8701) (6.6631, 2.9053) (6.6618, 2.9404) (6.6603, 2.9754) (6.6587, 3.0104) (6.6568, 3.0453) (6.6548, 3.0801) (6.6526, 3.1149) (6.6501, 3.1496) (6.6475, 3.1842) (6.6447, 3.2187) (6.6416, 3.2531) (6.6384, 3.2875) (6.6349, 3.3217) (6.6313, 3.3559) (6.6274, 3.39) (6.6234, 3.424) (6.6191, 3.4579) (6.6147, 3.4917) (6.61, 3.5254) (6.6051, 3.5591) (6.6, 3.5926) (6.5947, 3.626) (6.5891, 3.6593) (6.5834, 3.6926) (6.5774, 3.7257) (6.5713, 3.7587) (6.5649, 3.7916) (6.5582, 3.8243) (6.5514, 3.857) (6.5443, 3.8896) (6.5369, 3.922) (6.5294, 3.9543) (6.5216, 3.9865) (6.5136, 4.0185) (6.5053, 4.0505) (6.4968, 4.0822) (6.4881, 4.1139) (6.4791, 4.1454) (6.4698, 4.1768) (6.4602, 4.2079) (6.4504, 4.239) (6.4403, 4.2699) (6.4299, 4.3006) (6.4194, 4.3312) (6.4085, 4.3616) (6.3974, 4.3919) (6.3859, 4.4219) (6.3741, 4.4517) (6.3618, 4.4813) (6.3491, 4.5105) (6.336, 4.5396) (6.3226, 4.5684) (6.3091, 4.5971) (6.2953, 4.6257) (6.2813, 4.654) (6.2667, 4.682) (6.2513, 4.7095) (6.238, 4.7307) (6.2274, 4.7463) (6.22, 4.7564) (6.2162, 4.7615) knots -1 -1 -1 -1 -1 -1 -0.98571429 -0.97142857 -0.95714286 -0.94285714 -0.92857143 -0.91428571 -0.9 -0.88571429 -0.87142857 -0.85714286 -0.84285714 -0.82857143 -0.81428571 -0.8 -0.78571429 -0.77142857 -0.75714286 -0.74285714 -0.72857143 -0.71428571 -0.7 -0.68571429 -0.67142857 -0.65714286 -0.64285714 -0.62857143 -0.61428571 -0.6 -0.58571429 -0.57142857 -0.55714286 -0.54285714 -0.52857143 -0.51428571 -0.5 -0.48571429 -0.47142857 -0.45714286 -0.44285714 -0.42857143 -0.41428571 -0.4 -0.38571429 -0.37142857 -0.35714286 -0.34285714 -0.32857143 -0.31428571 -0.3 -0.28571429 -0.27142857 -0.25714286 -0.24285714 -0.22857143 -0.21428571 -0.2 -0.18571429 -0.17142857 -0.15714286 -0.14285714 -0.12857143 -0.11428571 -0.1 -0.08571429 -0.07142857 -0.05714286 -0.04285714 -0.02857143 -0.01428571 0 0 0 0 0 0
  line L11 (6.2162, 4.7615) -> (6.0555, 4.9759)
  arc A24 (6.1668, 6.0559) -> (6.0555, 4.9759) centre (6.6957, 5.4557) ccw
  arc A25 (6.1668, 6.0559) -> (6.3157, 6.1901) centre (0, 13.0546) ccw
  arc A26 (7.4015, 6.1878) -> (6.3157, 6.1901) centre (6.8574, 5.6013) ccw
  line L12 (7.4015, 6.1878) -> (7.5979, 6.0055)
  spline S12 degree 5 poles (7.5979, 6.0055) (7.6025, 6.0013) (7.6119, 5.9929) (7.6262, 5.9807) (7.646, 5.9652) (7.6717, 5.947) (7.698, 5.9296) (7.7247, 5.9127) (7.7517, 5.8961) (7.7788, 5.8796) (7.8061, 5.8633) (7.8336, 5.8472) (7.8614, 5.8315) (7.8895, 5.8162) (7.9179, 5.8013) (7.9465, 5.7867) (7.9755, 5.7725) (8.0046, 5.7586) (8.034, 5.7449) (8.0634, 5.7314) (8.0931, 5.7181) (8.1229, 5.7051) (8.1529, 5.6923) (8.1831, 5.6798) (8.2135, 5.6675) (8.2441, 5.6555) (8.2748, 5.6437) (8.3057, 5.6322) (8.3368, 5.6209) (8.368, 5.6098) (8.3993, 5.5989) (8.4308, 5.5882) (8.4624, 5.5777) (8.4942, 5.5675) (8.5261, 5.5575) (8.5581, 5.5477) (8.5903, 5.5381) (8.6226, 5.5287) (8.6551, 5.5195) (8.6876, 5.5105) (8.7203, 5.5017) (8.7531, 5.4931) (8.786, 5.4848) (8.8191, 5.4766) (8.8522, 5.4686) (8.8855, 5.4608) (8.9189, 5.4532) (8.9524, 5.4458) (8.986, 5.4387) (9.0197, 5.4317) (9.0536, 5.4248) (9.0875, 5.4182) (9.1215, 5.4118) (9.1556, 5.4056) (9.1899, 5.3995) (9.2242, 5.3936) (9.2586, 5.388) (9.2931, 5.3825) (9.3278, 5.3772) (9.3625, 5.3721) (9.3973, 5.3672) (9.4322, 5.3624) (9.4671, 5.3579) (9.5022, 5.3535) (9.5374, 5.3493) (9.5726, 5.3453) (9.6079, 5.3415) (9.6433, 5.3378) (9.6788, 5.3344) (9.7144, 5.3311) (9.75, 5.328) (9.7786, 5.3257) (9.8001, 5.324) (9.8144, 5.3229) (9.8216, 5.3224) knots 0 0 0 0 0 0 0.01428571 0.02857143 0.04285714 0.05714286 0.07142857 0.08571429 0.1 0.11428571 0.12857143 0.14285714 0.15714286 0.17142857 0.18571429 0.2 0.21428571 0.22857143 0.24285714 0.25714286 0.27142857 0.28571429 0.3 0.31428571 0.32857143 0.34285714 0.35714286 0.37142857 0.38571429 0.4 0.41428571 0.42857143 0.44285714 0.45714286 0.47142857 0.48571429 0.5 0.51428571 0.52857143 0.54285714 0.55714286 0.57142857 0.58571429 0.6 0.61428571 0.62857143 0.64285714 0.65714286 0.67142857 0.68571429 0.7 0.71428571 0.72857143 0.74285714 0.75714286 0.77142857 0.78571429 0.8 0.81428571 0.82857143 0.84285714 0.85714286 0.87142857 0.88571429 0.9 0.91428571 0.92857143 0.94285714 0.95714286 0.97142857 0.98571429 1 1 1 1 1 1
  arc A27 (9.8216, 5.3224) -> (10.3888, 6.1031) centre (0, 13.0546) ccw
  spline S13 degree 5 poles (10.3888, 6.1031) (10.3861, 6.1098) (10.3806, 6.1231) (10.3724, 6.143) (10.3614, 6.1694) (10.3474, 6.2024) (10.3333, 6.2352) (10.319, 6.2679) (10.3046, 6.3004) (10.2901, 6.3328) (10.2754, 6.3651) (10.2605, 6.3973) (10.2455, 6.4292) (10.2304, 6.4611) (10.2151, 6.4928) (10.1997, 6.5244) (10.1841, 6.5558) (10.1684, 6.5871) (10.1525, 6.6182) (10.1364, 6.6492) (10.1203, 6.6801) (10.1039, 6.7108) (10.0875, 6.7413) (10.0708, 6.7717) (10.054, 6.8019) (10.0371, 6.832) (10.02, 6.8619) (10.0028, 6.8916) (9.9854, 6.9212) (9.9679, 6.9506) (9.9502, 6.9798) (9.9324, 7.0089) (9.9144, 7.0378) (9.8962, 7.0665) (9.8779, 7.0951) (9.8595, 7.1235) (9.8409, 7.1516) (9.8221, 7.1797) (9.8032, 7.2075) (9.7841, 7.2351) (9.7649, 7.2626) (9.7455, 7.2898) (9.726, 7.3169) (9.7062, 7.3437) (9.6864, 7.3703) (9.6663, 7.3968) (9.6461, 7.423) (9.6258, 7.449) (9.6052, 7.4749) (9.5845, 7.5004) (9.5637, 7.5258) (9.5426, 7.5509) (9.5214, 7.5758) (9.5, 7.6004) (9.4783, 7.6247) (9.4566, 7.6488) (9.4346, 7.6727) (9.4125, 7.6964) (9.3902, 7.7198) (9.3678, 7.7429) (9.3451, 7.7657) (9.3221, 7.7881) (9.2989, 7.81) (9.2753, 7.8316) (9.2516, 7.8528) (9.2276, 7.8737) (9.2036, 7.8944) (9.1794, 7.9149) (9.1551, 7.9351) (9.1304, 7.9548) (9.1051, 7.9736) (9.0843, 7.9876) (9.0683, 7.9975) (9.0574, 8.0038) (9.0519, 8.0068) knots -1 -1 -1 -1 -1 -1 -0.98571429 -0.97142857 -0.95714286 -0.94285714 -0.92857143 -0.91428571 -0.9 -0.88571429 -0.87142857 -0.85714286 -0.84285714 -0.82857143 -0.81428571 -0.8 -0.78571429 -0.77142857 -0.75714286 -0.74285714 -0.72857143 -0.71428571 -0.7 -0.68571429 -0.67142857 -0.65714286 -0.64285714 -0.62857143 -0.61428571 -0.6 -0.58571429 -0.57142857 -0.55714286 -0.54285714 -0.52857143 -0.51428571 -0.5 -0.48571429 -0.47142857 -0.45714286 -0.44285714 -0.42857143 -0.41428571 -0.4 -0.38571429 -0.37142857 -0.35714286 -0.34285714 -0.32857143 -0.31428571 -0.3 -0.28571429 -0.27142857 -0.25714286 -0.24285714 -0.22857143 -0.21428571 -0.2 -0.18571429 -0.17142857 -0.15714286 -0.14285714 -0.12857143 -0.11428571 -0.1 -0.08571429 -0.07142857 -0.05714286 -0.04285714 -0.02857143 -0.01428571 0 0 0 0 0 0
  line L13 (9.0519, 8.0068) -> (8.8179, 8.1373)
  arc A28 (8.4802, 9.1693) -> (8.8179, 8.1373) centre (9.2075, 8.836) ccw
  arc A29 (8.4802, 9.1693) -> (8.5618, 9.3524) centre (0, 13.0546) ccw
  arc A30 (9.5546, 9.7919) -> (8.5618, 9.3524) centre (9.2961, 9.0348) ccw
  line L14 (9.5546, 9.7919) -> (9.8082, 9.7053)
  spline S14 degree 5 poles (9.8082, 9.7053) (9.8141, 9.7033) (9.8261, 9.6994) (9.8441, 9.6941) (9.8685, 9.6881) (9.8993, 9.6819) (9.9304, 9.6767) (9.9617, 9.6721) (9.9932, 9.6678) (10.0246, 9.6638) (10.0562, 9.66) (10.0879, 9.6566) (10.1196, 9.6535) (10.1515, 9.6509) (10.1835, 9.6489) (10.2156, 9.6472) (10.2479, 9.646) (10.2802, 9.6451) (10.3125, 9.6445) (10.345, 9.6442) (10.3774, 9.6441) (10.41, 9.6444) (10.4426, 9.6449) (10.4753, 9.6457) (10.508, 9.6469) (10.5409, 9.6484) (10.5737, 9.6501) (10.6066, 9.6521) (10.6396, 9.6544) (10.6726, 9.657) (10.7057, 9.6598) (10.7388, 9.6628) (10.7719, 9.6661) (10.8051, 9.6697) (10.8383, 9.6735) (10.8716, 9.6776) (10.9049, 9.6819) (10.9382, 9.6865) (10.9716, 9.6913) (11.005, 9.6963) (11.0384, 9.7016) (11.0719, 9.7071) (11.1054, 9.7128) (11.1389, 9.7188) (11.1724, 9.725) (11.206, 9.7314) (11.2396, 9.7381) (11.2732, 9.7449) (11.3068, 9.752) (11.3405, 9.7593) (11.3741, 9.7669) (11.4078, 9.7746) (11.4415, 9.7826) (11.4752, 9.7908) (11.509, 9.7992) (11.5427, 9.8078) (11.5765, 9.8166) (11.6102, 9.8256) (11.644, 9.8349) (11.6778, 9.8443) (11.7116, 9.854) (11.7454, 9.8639) (11.7792, 9.8739) (11.813, 9.8842) (11.8468, 9.8947) (11.8807, 9.9053) (11.9145, 9.9162) (11.9483, 9.9273) (11.9821, 9.9386) (12.0159, 9.95) (12.0498, 9.9617) (12.0768, 9.9712) (12.0971, 9.9784) (12.1106, 9.9832) (12.1174, 9.9857) knots 0 0 0 0 0 0 0.01428571 0.02857143 0.04285714 0.05714286 0.07142857 0.08571429 0.1 0.11428571 0.12857143 0.14285714 0.15714286 0.17142857 0.18571429 0.2 0.21428571 0.22857143 0.24285714 0.25714286 0.27142857 0.28571429 0.3 0.31428571 0.32857143 0.34285714 0.35714286 0.37142857 0.38571429 0.4 0.41428571 0.42857143 0.44285714 0.45714286 0.47142857 0.48571429 0.5 0.51428571 0.52857143 0.54285714 0.55714286 0.57142857 0.58571429 0.6 0.61428571 0.62857143 0.64285714 0.65714286 0.67142857 0.68571429 0.7 0.71428571 0.72857143 0.74285714 0.75714286 0.77142857 0.78571429 0.8 0.81428571 0.82857143 0.84285714 0.85714286 0.87142857 0.88571429 0.9 0.91428571 0.92857143 0.94285714 0.95714286 0.97142857 0.98571429 1 1 1 1 1 1
  arc A31 (12.1174, 9.9857) -> (12.3181, 10.9296) centre (0, 13.0546) ccw
  spline S15 degree 5 poles (12.3181, 10.9296) (12.3129, 10.9346) (12.3025, 10.9445) (12.2869, 10.9594) (12.266, 10.979) (12.2399, 11.0035) (12.2136, 11.0277) (12.1873, 11.0518) (12.1609, 11.0756) (12.1344, 11.0993) (12.1079, 11.1228) (12.0813, 11.1461) (12.0545, 11.1693) (12.0278, 11.1922) (12.0009, 11.215) (11.9739, 11.2375) (11.9469, 11.2599) (11.9198, 11.2821) (11.8926, 11.3041) (11.8654, 11.3259) (11.8381, 11.3475) (11.8107, 11.3689) (11.7832, 11.39) (11.7557, 11.411) (11.728, 11.4318) (11.7003, 11.4524) (11.6726, 11.4728) (11.6447, 11.4929) (11.6168, 11.5129) (11.5889, 11.5326) (11.5608, 11.5521) (11.5327, 11.5714) (11.5045, 11.5905) (11.4762, 11.6094) (11.4479, 11.628) (11.4195, 11.6464) (11.3911, 11.6646) (11.3625, 11.6826) (11.3339, 11.7003) (11.3053, 11.7178) (11.2765, 11.7351) (11.2477, 11.7521) (11.2189, 11.7688) (11.1899, 11.7853) (11.1609, 11.8016) (11.1319, 11.8176) (11.1027, 11.8333) (11.0736, 11.8488) (11.0443, 11.8641) (11.015, 11.879) (10.9856, 11.8937) (10.9562, 11.9081) (10.9267, 11.9221) (10.8971, 11.9359) (10.8674, 11.9494) (10.8377, 11.9625) (10.808, 11.9754) (10.7782, 11.988) (10.7483, 12.0003) (10.7184, 12.0123) (10.6883, 12.0239) (10.6583, 12.035) (10.6281, 12.0457) (10.5978, 12.0558) (10.5675, 12.0655) (10.5371, 12.0749) (10.5067, 12.084) (10.4763, 12.0929) (10.4458, 12.1014) (10.4153, 12.1093) (10.3846, 12.1162) (10.3599, 12.1206) (10.3412, 12.1231) (10.3287, 12.1244) (10.3225, 12.125) knots -1 -1 -1 -1 -1 -1 -0.98571429 -0.97142857 -0.95714286 -0.94285714 -0.92857143 -0.91428571 -0.9 -0.88571429 -0.87142857 -0.85714286 -0.84285714 -0.82857143 -0.81428571 -0.8 -0.78571429 -0.77142857 -0.75714286 -0.74285714 -0.72857143 -0.71428571 -0.7 -0.68571429 -0.67142857 -0.65714286 -0.64285714 -0.62857143 -0.61428571 -0.6 -0.58571429 -0.57142857 -0.55714286 -0.54285714 -0.52857143 -0.51428571 -0.5 -0.48571429 -0.47142857 -0.45714286 -0.44285714 -0.42857143 -0.41428571 -0.4 -0.38571429 -0.37142857 -0.35714286 -0.34285714 -0.32857143 -0.31428571 -0.3 -0.28571429 -0.27142857 -0.25714286 -0.24285714 -0.22857143 -0.21428571 -0.2 -0.18571429 -0.17142857 -0.15714286 -0.14285714 -0.12857143 -0.11428571 -0.1 -0.08571429 -0.07142857 -0.05714286 -0.04285714 -0.02857143 -0.01428571 0 0 0 0 0 0
  line L15 (10.3225, 12.125) -> (10.0556, 12.149)
  arc A32 (9.3274, 12.9544) -> (10.0556, 12.149) centre (10.1274, 12.9458) ccw
  arc A33 (9.3274, 12.9544) -> (9.3274, 13.1548) centre (0, 13.0546) ccw
  arc A34 (10.0556, 13.9602) -> (9.3274, 13.1548) centre (10.1274, 13.1634) ccw
  line L16 (10.0556, 13.9602) -> (10.3225, 13.9842)
  spline S16 degree 5 poles (10.3225, 13.9842) (10.3287, 13.9848) (10.3412, 13.9861) (10.3599, 13.9886) (10.3846, 13.993) (10.4153, 13.9999) (10.4458, 14.0078) (10.4763, 14.0163) (10.5067, 14.0252) (10.5371, 14.0344) (10.5675, 14.0437) (10.5978, 14.0534) (10.6281, 14.0636) (10.6583, 14.0742) (10.6883, 14.0853) (10.7184, 14.0969) (10.7483, 14.1089) (10.7782, 14.1212) (10.808, 14.1338) (10.8377, 14.1467) (10.8674, 14.1599) (10.8971, 14.1733) (10.9267, 14.1871) (10.9562, 14.2011) (10.9856, 14.2155) (11.015, 14.2302) (11.0443, 14.2452) (11.0736, 14.2604) (11.1027, 14.2759) (11.1319, 14.2916) (11.1609, 14.3076) (11.1899, 14.3239) (11.2189, 14.3404) (11.2477, 14.3572) (11.2765, 14.3742) (11.3053, 14.3914) (11.3339, 14.4089) (11.3625, 14.4266) (11.3911, 14.4446) (11.4195, 14.4628) (11.4479, 14.4812) (11.4762, 14.4998) (11.5045, 14.5187) (11.5327, 14.5378) (11.5608, 14.5571) (11.5889, 14.5766) (11.6168, 14.5963) (11.6447, 14.6163) (11.6726, 14.6365) (11.7003, 14.6568) (11.728, 14.6774) (11.7557, 14.6982) (11.7832, 14.7192) (11.8107, 14.7404) (11.8381, 14.7618) (11.8654, 14.7833) (11.8926, 14.8051) (11.9198, 14.8271) (11.9469, 14.8493) (11.9739, 14.8717) (12.0009, 14.8942) (12.0278, 14.917) (12.0545, 14.9399) (12.0813, 14.9631) (12.1079, 14.9864) (12.1344, 15.0099) (12.1609, 15.0336) (12.1873, 15.0575) (12.2136, 15.0815) (12.2399, 15.1058) (12.266, 15.1302) (12.2869, 15.1499) (12.3025, 15.1647) (12.3129, 15.1746) (12.3181, 15.1796) knots 0 0 0 0 0 0 0.01428571 0.02857143 0.04285714 0.05714286 0.07142857 0.08571429 0.1 0.11428571 0.12857143 0.14285714 0.15714286 0.17142857 0.18571429 0.2 0.21428571 0.22857143 0.24285714 0.25714286 0.27142857 0.28571429 0.3 0.31428571 0.32857143 0.34285714 0.35714286 0.37142857 0.38571429 0.4 0.41428571 0.42857143 0.44285714 0.45714286 0.47142857 0.48571429 0.5 0.51428571 0.52857143 0.54285714 0.55714286 0.57142857 0.58571429 0.6 0.61428571 0.62857143 0.64285714 0.65714286 0.67142857 0.68571429 0.7 0.71428571 0.72857143 0.74285714 0.75714286 0.77142857 0.78571429 0.8 0.81428571 0.82857143 0.84285714 0.85714286 0.87142857 0.88571429 0.9 0.91428571 0.92857143 0.94285714 0.95714286 0.97142857 0.98571429 1 1 1 1 1 1
  arc A35 (12.3181, 15.1796) -> (12.1174, 16.1235) centre (0, 13.0546) ccw